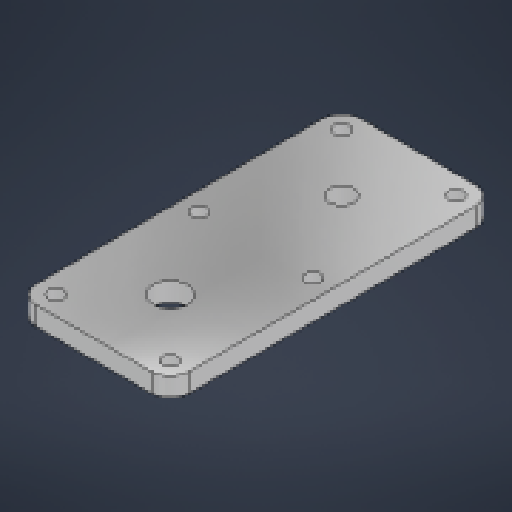
# Autodesk Inventor part: PLATE,MAGNET-MOUNT
Saved by Autodesk Inventor 2026.1 (Build 301233020, 233B)
## iProperties
Created: 2026-03-20
Part Number: PLATE,MAGNET-MOUNT
Material: Aluminum 6061
Document SubType Name: Sheet Metal
Designer: Owen L
Density: 2.7 g/cm^3
Sheet Metal Rule: Default
Appearance: Aluminum - Flat
Author: Owen L
Autodesk Inventor part; units mm, degrees
ref_plane "YZ Plane" through (0, 0, 0) normal (1, 0, 0) x (0, 1, 0)
ref_plane "XZ Plane" through (0, 0, 0) normal (0, 1, 0) x (-1, 0, 0)
ref_plane "XY Plane" through (0, 0, 0) normal (0, 0, 1) x (1, 0, 0)
sketch "Sketch1" plane through (0, 0, 0) normal (0, 1, 0) x (-1, 0, 0)
  line L0 (25.4, 60.325) -> (-25.4, 60.325)
  line L1 (-25.4, 60.325) -> (-25.4, -60.325)
  line L2 (-25.4, -60.325) -> (25.4, -60.325)
  line L3 (25.4, -60.325) -> (25.4, 60.325)
  line L4 (25.4, 60.325) -> (-25.4, -60.325) construction
  line L5 (-25.4, 60.325) -> (25.4, -60.325) construction
  point P0 (0, 0)
  point P1 (0, 28.575)
  point P2 (0, -28.575)
  dimension "d0" = 50.8
  dimension "d1" = 120.65
  dimension "d2" = 57.15
  dimension "d3" = 28.575
  measures "d0" distance of L1.end L2.end
  measures "d1" distance of L0.end L1.end
  measures "d2" distance of point (0, 28.575) point (0, -28.575)
  measures "d3" distance of point (0, 0) point (0, 28.575)
extrude "Plate1" add sketch "Sketch1" along normal blind 6.35
sketch "Sketch2" plane through (0, 0, 0) normal (0, -1, 0) x (1, 0, 0)
  circle A0 centre (0, 28.575) radius 5.715
  circle A1 centre (0, -28.575) radius 4.1
  point P0 (0, 0)
  dimension "d5" = 28.575
  dimension "d6" = 11.43
  dimension "d9" = 28.575
  dimension "d10" = 8.2
  constraints: 2 centre point, 2 coincident, 2 vertical alignment
  measures "d5" distance of point (0, 0) point (0, 28.575)
  measures "d6" diameter of A0
  measures "d9" distance of point (0, 0) point (0, -28.575)
  measures "d10" diameter of A1
extrude "Cut1" cut sketch "Sketch2" against normal blind 6.35
sketch "Sketch3" plane through (0, 0, 0) normal (0, -1, 0) x (1, 0, 0)
  line L0 (-25.4, 60.325) -> (25.4, 60.325) construction
  line L1 (-25.4, -60.325) -> (-25.4, 60.325) construction
  circle A0 centre (0, 28.575) radius 5.715 projected
  circle A1 centre (0, 28.575) radius 25.4 construction
  circle A2 centre (0, -28.575) radius 4.1 projected
  circle A3 centre (0, -28.575) radius 25.4 construction
  point P0 (0, 0)
  point P1 (-19.05, 53.975)
  point P2 (19.05, 53.975)
  point P3 (-19.05, 0)
  point P4 (19.05, 0)
  point P5 (-19.05, -53.975)
  point P6 (19.05, -53.975)
  dimension "d13" = 38.1
  dimension "d16" = 53.975
  dimension "d19" = 6.35
  dimension "d20" = 6.35
  dimension "d29" = 50.8
  dimension "d30" = 50.8
  constraints: 2 centre point, 2 coincident, 1 horizontal, 1 vertical, 5 other
  measures "d13" distance of point (-19.05, 53.975) point (19.05, 53.975)
  measures "d16" distance of point (-19.05, 53.975) point (-19.05, 0)
  measures "d19" distance from line of L1 point (-19.05, 53.975)
  measures "d20" distance from line of L0 point (-19.05, 53.975)
  measures "d29" diameter of A1
  measures "d30" diameter of A3
hole "Hole1" at (-19.05, 0, 53.975) at (19.05, 0, 53.975) at (-19.05, 0, 0) at (19.05, 0, 0) at (-19.05, 0, -53.975) at (19.05, 0, -53.975) direction (0, 1, 0) diameter 5.1054 end through all clearance for "Flat Head Machine Screw (82)" size "#10" standard "Ansi Unified Screw Threads"
fillet "Corner Round1" radius 6.35 4 edges at (25.4, 3.175, -60.325) (-25.4, 3.175, -60.325) (25.4, 3.175, 60.325) (-25.4, 3.175, 60.325)
equation "\"d9\" = d5"
equation "\"d7\" = Thickness"
equation "\"d26\" = Thickness"
equation "\"d4\" = Thickness"
equation "\"BendRadius\" = Thickness"
equation "\"BendReliefWidth\" = Thickness"
equation "\"BendReliefDepth\" = 0.5 * Thickness"
equation "\"CornerReliefSize\" = 4 * Thickness"
equation "\"MinimumRemnant\" = 2 * Thickness"
equation "\"TransitionRadius\" = BendRadius"
equation "\"JacobiRadiusSize\" = BendRadius"
equation "\"GapSize\" = Thickness"
equation "\"Thickness\" = 6.35"
body "Solid1"
